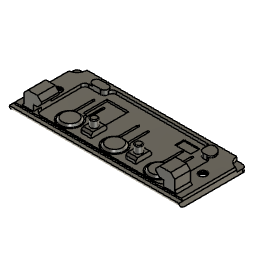
P3_Clicker (Autodesk Fusion 360 design; units mm, degrees)
Autodesk Fusion 360 part; units mm, degrees
sketch "草图1" plane through (0, 0, 0) normal (0, 0, 1) x (1, 0, 0)
  line L0 (0, 0) -> (43, 0)
  line L1 (43, 0) -> (43, 17.2)
  line L2 (43, 17.2) -> (0, 17.2)
  line L3 (0, 17.2) -> (0, 0)
  line L4 (0, 17.2) -> (3.1, 17.2) construction
  line L5 (3.1, 17.2) -> (3.1, 9.2) construction
  line L6 (3.1, 9.2) -> (0, 9.2) construction
  line L7 (0, 9.2) -> (0, 17.2) construction
  line L8 (21.5, 17.2) -> (21.5, 0) construction
  circle A0 centre (3.1, 9.2) radius 1.025
  circle A1 centre (3.1, 9.2) radius 2.05
  circle A2 centre (39.9, 9.2) radius 1.025
  circle A3 centre (39.9, 9.2) radius 2.05
  dimension "d1" = 43
  dimension "d2" = 17.2
  dimension "d17" = 3.1
  dimension "d18" = 8
  dimension "d19" = 2.05
  dimension "d20" = 4.1
  constraint horizontal L0
  constraint vertical L1
  constraint horizontal L2
  constraint vertical L3
  constraint coincident L0.start L3.end
  constraint horizontal L4
  constraint vertical L5
  constraint horizontal L6
  constraint vertical L7
  constraint midpoint L2 L8.start
  constraint midpoint L0 L8.end
  constraint coincident L5.end L6.start
  constraint concentric A0 A1
  constraint symmetric L8 A0 A2
  constraint symmetric L8 A1 A3
  measures "d1" distance of L0.start L0.end
  measures "d2" distance of L0.start L2.end
  measures "d17" distance of L2.end L4.end
  measures "d18" distance of L2.end L6.end
  measures "d19" diameter of A0
  measures "d20" diameter of A1
extrude "拉伸1" add sketch "草图1" along normal blind 1.8 contours L0 L1 L2 L3 | A0 | A1 | A2 | A3
sketch "草图2" plane through (0, 0, 1.8) normal (0, 0, 1) x (-1, 0, 0)
  line L0 (0, -17.2) -> (0, 0)
  line L1 (0, 0) -> (-43, 0)
  line L2 (-43, 0) -> (-43, -17.2)
  line L3 (-43, -17.2) -> (0, -17.2)
  circle A0 centre (0, -17.2) radius 2.5
  circle A1 centre (-43, -17.2) radius 2.5
  line L4 (0, 0) -> (-43, 0)
  line L5 (-43, 0) -> (-43, -1)
  line L6 (-43, -1) -> (0, -1)
  line L7 (0, -1) -> (0, 0)
  dimension "d5" = 5
  dimension "d6" = 5
  dimension "d11" = 1
  constraint coincident L0.start L3.end
  constraint coincident L2.end L3.start
  constraint horizontal L4
  constraint vertical L5
  constraint horizontal L6
  constraint vertical L7
  constraint coincident L0.end L1.start
  measures "d5" diameter of A0
  measures "d6" diameter of A1
  measures "d11" distance of L0.end L6.end
extrude "拉伸2" cut sketch "草图2" against normal blind 0.9 contours L0 L3 A0 | L2 L3 A1 picked at (-1.3308, -16.2037) picked at (-41.5409, -16.4033)
fillet "圆角1" radius 1 2 edges at (43, 17.2, 0.45) (0, 17.2, 0.45)
extrude "拉伸3" cut sketch "草图2" against normal blind 0.4 contours L0 L1 L2 L4 L5 L6 L7
fillet "圆角3" radius 1.5 1 edges at (21.5, 0, 0)
chamfer "倒角1" distance 0.4 angle 45 2 edges at (43, 7.85, 1.8) (0, 7.85, 1.8)
extrude "拉伸4" cut sketch "草图1" along normal up to surface (1.8 mm away) contours A0 | A2
extrude "拉伸5" cut sketch "草图1" along normal blind 0.5 contours A1 | A3
chamfer "倒角3" distance 1 angle 45 2 edges at (38.9444, 9.5707, 0.5) (2.1444, 9.5707, 0.5)
chamfer "倒角4" distance 0.2 angle 45 2 edges at (1.1887, 8.4587, 0) (37.9887, 8.4587, 0)
sketch "草图3" plane through (0, 0, 0) normal (0, 0, 1) x (1, 0, 0)
  line L0 (43, 17.2) -> (0, 17.2)
  line L1 (0, 17.2) -> (0, 0)
  line L2 (0, 0) -> (43, 0)
  line L3 (43, 0) -> (43, 17.2)
  circle A0 centre (3.1, 9.2) radius 2.05
  circle A1 centre (3.1, 9.2) radius 1.025
  circle A2 centre (39.9, 9.2) radius 2.05
  circle A3 centre (39.9, 9.2) radius 1.025
  line L4 (3.1, 9.2) -> (0, 9.2) construction
  line L5 (3.1, 17.2) -> (3.1, 9.2) construction
  line L6 (0, 9.2) -> (43, 9.2) construction
  line L7 (21.5, 16.2) -> (21.5, 18) construction
  line L8 (5.5, 9.2) -> (37.5, 9.2) construction
  line L9 (21.5, 17.2) -> (21.5, 0) construction
  line L10 (6.7892, 15.8535) -> (35.7892, 15.8535) construction
  line L11 (37.2892, 14.3535) -> (37.2892, 3.3535) construction
  line L12 (35.7892, 1.8535) -> (6.7892, 1.8535) construction
  line L13 (5.2892, 3.3535) -> (5.2892, 14.3535) construction
  line L14 (5.2892, 8.6) -> (37.2892, 8.6) construction
  line L15 (22.2892, 15.8535) -> (22.2892, 1.8535) construction
  line L16 (0, 8.6) -> (43, 8.6) construction
  arc A4 (6.7892, 15.8535) -> (5.2892, 14.3535) centre (6.7892, 14.3535) ccw construction
  arc A5 (5.2892, 3.3535) -> (6.7892, 1.8535) centre (6.7892, 3.3535) ccw construction
  arc A6 (35.7892, 1.8535) -> (37.2892, 3.3535) centre (35.7892, 3.3535) ccw construction
  arc A7 (37.2892, 14.3535) -> (35.7892, 15.8535) centre (35.7892, 14.3535) ccw construction
  arc A8 (37.7892, 14.3535) -> (35.7892, 16.3535) centre (35.7892, 14.3535) ccw
  line L17 (6.7892, 16.3535) -> (35.7892, 16.3535)
  arc A9 (6.7892, 16.3535) -> (4.7892, 14.3535) centre (6.7892, 14.3535) ccw
  line L18 (4.7892, 3.3535) -> (4.7892, 14.3535)
  arc A10 (4.7892, 3.3535) -> (6.7892, 1.3535) centre (6.7892, 3.3535) ccw
  line L19 (35.7892, 1.3535) -> (6.7892, 1.3535)
  arc A11 (35.7892, 1.3535) -> (37.7892, 3.3535) centre (35.7892, 3.3535) ccw
  line L20 (37.7892, 14.3535) -> (37.7892, 3.3535)
  point P0 (5.2892, 15.8535)
  point P1 (37.2892, 15.8535)
  point P2 (5.2892, 1.8535)
  dimension "d33" = 32
  dimension "d34" = 14
  dimension "d35" = 1.5
  dimension "d36" = 0.5
  constraint coincident L4.end L6.start
  constraint coincident L3 L6.end
  constraint perpendicular L3 L6
  constraint collinear L7 L9
  constraint horizontal L10
  constraint vertical L11
  constraint horizontal L12
  constraint vertical L13
  constraint midpoint L1 L16.start
  constraint midpoint L3 L16.end
  constraint collinear L14 L16
  constraint coincident L10 L15.start
  constraint coincident L13 L14.start
  constraint coincident P0 L10
  constraint coincident P0 L13
  constraint tangent L10 A4
  constraint tangent L13 A4
  constraint coincident L12 L15.end
  constraint coincident P2 L12
  constraint coincident P2 L13
  constraint tangent L12 A5
  constraint tangent L13 A5
  constraint equal A4 A5
  constraint coincident L11 L14.end
  constraint tangent L11 A6
  constraint tangent L12 A6
  constraint equal A4 A6
  constraint coincident P1 L10
  constraint coincident P1 L11
  constraint tangent L10 A7
  constraint tangent L11 A7
  constraint equal A4 A7
  measures "d33" distance of P0 P1
  measures "d34" distance of P0 P2
  measures "d35" radius of A4
sketch "草图4" plane through (0, 0, 1.8) normal (0, 0, 1) x (-1, 0, 0)
  circle A0 centre (-39.9, -9.2) radius 1.025
  circle A1 centre (-3.1, -9.2) radius 1.025
  line L0 (-0.4, -14.7322) -> (-0.4, -1)
  line L1 (-0.4, -1) -> (-42.6, -1)
  line L2 (-42.6, -1) -> (-42.6, -14.7322)
  arc A2 (-40.5, -17.2) -> (-42.6, -14.7322) centre (-43, -17.2) ccw
  line L3 (-40.5, -17.2) -> (-2.5, -17.2)
  arc A3 (-0.4, -14.7322) -> (-2.5, -17.2) centre (0, -17.2) ccw
  arc A4 (-37.7892, -14.3535) -> (-35.7892, -16.3535) centre (-35.7892, -14.3535) ccw
  line L4 (-37.7892, -14.3535) -> (-37.7892, -3.3535)
  arc A5 (-35.7892, -1.3535) -> (-37.7892, -3.3535) centre (-35.7892, -3.3535) ccw
  line L5 (-35.7892, -1.3535) -> (-6.7892, -1.3535)
  arc A6 (-4.7892, -3.3535) -> (-6.7892, -1.3535) centre (-6.7892, -3.3535) ccw
  line L6 (-4.7892, -3.3535) -> (-4.7892, -14.3535)
  arc A7 (-6.7892, -16.3535) -> (-4.7892, -14.3535) centre (-6.7892, -14.3535) ccw
  line L7 (-6.7892, -16.3535) -> (-35.7892, -16.3535)
  line L8 (-10.6464, -14.1527) -> (-16.1464, -14.1527)
  line L9 (-16.1464, -14.1527) -> (-16.1464, -8.1527)
  line L10 (-16.1464, -8.1527) -> (-10.6464, -8.1527)
  line L11 (-10.6464, -8.1527) -> (-10.6464, -14.1527)
  circle A8 centre (-16, -5.5) radius 0.9
  circle A9 centre (-27.3, -5.5) radius 0.9
  line L12 (-29.3027, -15.0275) -> (-33.3027, -15.0275)
  line L13 (-33.3027, -15.0275) -> (-33.3027, -12.7275)
  line L14 (-33.3027, -12.7275) -> (-29.3027, -12.7275)
  line L15 (-29.3027, -12.7275) -> (-29.3027, -15.0275)
  dimension "d39" = 5.5
  dimension "d40" = 6
  dimension "d43" = 1.8
  dimension "d44" = 1.8
  dimension "d84" = 4
  dimension "d85" = 2.3
  constraint horizontal L8
  constraint vertical L9
  constraint horizontal L10
  constraint vertical L11
  constraint horizontal L12
  constraint vertical L13
  constraint horizontal L14
  constraint vertical L15
  measures "d39" distance of L8.start L8.end
  measures "d40" distance of L8.start L10.end
  measures "d43" diameter of A8
  measures "d44" diameter of A9
  measures "d84" distance of L12.start L12.end
  measures "d85" distance of L12.start L14.end
extrude "拉伸6" cut sketch "草图4" against normal blind 0.8 contours A4 L4 A5 L5 A6 L6 A7 L7 | L8 L9 L10 L11 | A8 | A9 | L12 L13 L14 L15
sketch "草图5" plane through (0, 0, 1) normal (0, 0, 1) x (-1, 0, 0)
  line L0 (-37.7892, -3.3535) -> (-37.7892, -14.3535)
  arc A0 (-37.7892, -14.3535) -> (-35.7892, -16.3535) centre (-35.7892, -14.3535) ccw
  line L1 (-35.7892, -16.3535) -> (-6.7892, -16.3535)
  arc A1 (-6.7892, -16.3535) -> (-4.7892, -14.3535) centre (-6.7892, -14.3535) ccw
  line L2 (-4.7892, -14.3535) -> (-4.7892, -3.3535)
  arc A2 (-4.7892, -3.3535) -> (-6.7892, -1.3535) centre (-6.7892, -3.3535) ccw
  line L3 (-6.7892, -1.3535) -> (-35.7892, -1.3535)
  arc A3 (-35.7892, -1.3535) -> (-37.7892, -3.3535) centre (-35.7892, -3.3535) ccw
  line L4 (-16.1464, -8.1527) -> (-10.6464, -8.1527)
  line L5 (-10.6464, -8.1527) -> (-10.6464, -14.1527)
  line L6 (-16.1464, -14.1527) -> (-16.1464, -8.1527)
  line L7 (-10.6464, -14.1527) -> (-16.1464, -14.1527)
  circle A4 centre (-16, -5.5) radius 0.9
  circle A5 centre (-27.3, -5.5) radius 0.9
  circle A6 centre (-21.6977, -5.0059) radius 2.5
  line L8 (-20.6977, -12.0059) -> (-22.6977, -12.0059)
  line L9 (-22.6977, -12.0059) -> (-22.6977, -5.0059)
  line L10 (-22.6977, -5.0059) -> (-20.6977, -5.0059)
  line L11 (-20.6977, -5.0059) -> (-20.6977, -12.0059)
  line L12 (-20.1977, -4.5059) -> (-20.1977, -12.5059)
  line L13 (-20.1977, -12.5059) -> (-23.1977, -12.5059)
  line L14 (-23.1977, -12.5059) -> (-23.1977, -4.5059)
  line L15 (-23.1977, -4.5059) -> (-20.1977, -4.5059)
  circle A7 centre (-21.6977, -5.0059) radius 2.8
  line L16 (-31.3977, -4.5059) -> (-31.3977, -12.5059)
  line L17 (-31.3977, -12.5059) -> (-34.3977, -12.5059)
  line L18 (-34.3977, -4.5059) -> (-31.3977, -4.5059)
  line L19 (-34.3977, -12.5059) -> (-34.3977, -4.5059)
  line L20 (-31.8977, -5.0059) -> (-31.8977, -12.0059)
  line L21 (-31.8977, -12.0059) -> (-33.8977, -12.0059)
  line L22 (-33.8977, -5.0059) -> (-31.8977, -5.0059)
  line L23 (-33.8977, -12.0059) -> (-33.8977, -5.0059)
  circle A8 centre (-32.8977, -5.0059) radius 2.8
  circle A9 centre (-32.8977, -5.0059) radius 2.5
  line L24 (-11.8977, -12.5059) -> (-11.8977, -4.5059)
  line L25 (-11.8977, -4.5059) -> (-8.8977, -4.5059)
  line L26 (-8.8977, -4.5059) -> (-8.8977, -12.5059)
  line L27 (-8.8977, -12.5059) -> (-11.8977, -12.5059)
  line L28 (-11.3977, -12.0059) -> (-11.3977, -5.0059)
  line L29 (-11.3977, -5.0059) -> (-9.3977, -5.0059)
  line L30 (-9.3977, -12.0059) -> (-11.3977, -12.0059)
  line L31 (-9.3977, -5.0059) -> (-9.3977, -12.0059)
  circle A10 centre (-10.3977, -5.0059) radius 2.8
  circle A11 centre (-10.3977, -5.0059) radius 2.5
  line L32 (-9.3977, -12.0059) -> (-9.3977, -12.5059)
  line L33 (-11.3977, -12.0059) -> (-11.3977, -12.5059)
  line L34 (-22.6977, -12.0059) -> (-22.6977, -12.5059)
  line L35 (-20.6977, -12.0059) -> (-20.6977, -12.5059)
  line L36 (-33.8977, -12.0059) -> (-33.8977, -12.5059)
  line L37 (-31.8977, -12.0059) -> (-31.8977, -12.5059)
  line L38 (-33.3027, -12.7275) -> (-29.3027, -12.7275)
  line L39 (-29.3027, -12.7275) -> (-29.3027, -15.0275)
  line L40 (-33.3027, -15.0275) -> (-33.3027, -12.7275)
  line L41 (-29.3027, -15.0275) -> (-33.3027, -15.0275)
  line L42 (-14.75, -7.5) -> (-17.25, -7.5)
  line L43 (-17.25, -7.5) -> (-17.25, -3.5)
  line L44 (-17.25, -3.5) -> (-14.75, -3.5)
  line L45 (-14.75, -3.5) -> (-14.75, -7.5)
  line L46 (-14.75, -7.5) -> (-17.25, -3.5) construction
  line L47 (-17.25, -7.5) -> (-14.75, -3.5) construction
  line L48 (-28.55, -7.5) -> (-26.05, -7.5)
  line L49 (-26.05, -7.5) -> (-26.05, -3.5)
  line L50 (-26.05, -3.5) -> (-28.55, -3.5)
  line L51 (-28.55, -3.5) -> (-28.55, -7.5)
  line L52 (-28.55, -7.5) -> (-26.05, -3.5) construction
  line L53 (-26.05, -7.5) -> (-28.55, -3.5) construction
  line L54 (-4.7892, -16.3535) -> (-9.7892, -16.3535)
  line L55 (-9.7892, -16.3535) -> (-9.7892, -14.3535)
  line L56 (-9.7892, -14.3535) -> (-4.7892, -14.3535)
  line L57 (-4.7892, -14.3535) -> (-4.7892, -16.3535)
  line L58 (-37.7892, -16.3535) -> (-34.7892, -16.3535)
  line L59 (-34.7892, -16.3535) -> (-34.7892, -13.3535)
  line L60 (-34.7892, -13.3535) -> (-37.7892, -13.3535)
  line L61 (-37.7892, -13.3535) -> (-37.7892, -16.3535)
  point P0 (-16, -5.5)
  point P1 (-27.3, -5.5)
  dimension "d46" = 5
  dimension "d53" = 2
  dimension "d54" = 7
  dimension "d58" = -0.5
  dimension "d59" = 0.3
  dimension "d60" = -0.5
  dimension "d61" = 0.3
  dimension "d62" = 5
  dimension "d63" = 2
  dimension "d64" = 7
  dimension "d65" = -0.5
  dimension "d66" = 0.3
  dimension "d67" = 5
  dimension "d68" = 2
  dimension "d69" = 7
  dimension "d151" = 1.8
  dimension "d152" = 1.8
  dimension "d156" = 2.5
  dimension "d157" = 4
  dimension "d158" = 2.5
  dimension "d159" = 4
  dimension "d163" = 5
  dimension "d164" = 2
  dimension "d165" = 3
  dimension "d166" = 3
  constraint horizontal L8
  constraint vertical L9
  constraint horizontal L10
  constraint vertical L11
  constraint midpoint A6.centre L10
  constraint horizontal L21
  constraint vertical L23
  constraint horizontal L22
  constraint vertical L20
  constraint midpoint A8.centre L22
  constraint horizontal L30
  constraint vertical L28
  constraint horizontal L29
  constraint vertical L31
  constraint midpoint A10.centre L29
  constraint coincident L27 L32.end
  constraint perpendicular L27 L32
  constraint coincident L27 L33.end
  constraint perpendicular L27 L33
  constraint coincident L13 L34.end
  constraint perpendicular L13 L34
  constraint coincident L13 L35.end
  constraint perpendicular L13 L35
  constraint coincident L17 L36.end
  constraint perpendicular L17 L36
  constraint coincident L17 L37.end
  constraint perpendicular L17 L37
  constraint collinear L13 L27
  constraint collinear L13 L17
  constraint horizontal L42
  constraint perpendicular L42 L43
  constraint parallel L42 L44
  constraint parallel L43 L45
  constraint coincident L46 P0
  constraint coincident L47 P0
  constraint coincident P0 A4.centre
  constraint horizontal L48
  constraint perpendicular L48 L49
  constraint parallel L48 L50
  constraint parallel L49 L51
  constraint coincident L52 P1
  constraint coincident L53 P1
  constraint coincident P1 A5.centre
  constraint horizontal L54
  constraint vertical L55
  constraint horizontal L56
  constraint vertical L57
  constraint horizontal L58
  constraint vertical L59
  constraint horizontal L60
  constraint vertical L61
  measures "d46" diameter of A6
  measures "d53" distance of L8.start L8.end
  measures "d54" distance of L8.start L10.end
  measures "d62" diameter of A9
  measures "d63" distance of L20.end L21.end
  measures "d64" distance of L20.start L20.end
  measures "d67" diameter of A11
  measures "d68" distance of L30.start L28.start
  measures "d69" distance of L29.end L30.start
  measures "d151" diameter of A4
  measures "d152" diameter of A5
  measures "d156" distance of L43.end L44.end
  measures "d157" distance of L42.end L43.end
  measures "d158" distance of L49.end L50.end
  measures "d159" distance of L48.end L49.end
  measures "d163" distance of L54.start L54.end
  measures "d164" distance of L54.start A1.end
  measures "d165" distance of L58.start L58.end
  measures "d166" distance of L58.start L60.end
extrude "拉伸21" add sketch "草图5" along normal blind 1.2 contours L0 A0 L1 L58 L59 L60 L61 | L1 A1 L54 L55 L56
fillet "圆角9" radius 1 10 edges at (9.7892, 14.3535, 1.6) (34.7892, 13.3535, 1.6) (9.7892, 16.3535, 1.4) (4.7892, 14.3535, 1.4) (37.7892, 13.3535, 1.4) (34.7892, 16.3535, 1.4) (4.7892, 14.3535, 2) (9.7892, 16.3535, 2) (37.7892, 13.3535, 2) (34.7892, 16.3535, 2)
extrude "拉伸20" add sketch "草图5" along normal blind 1.2 contours L42 L43 L44 L45 | L48 L49 L50 L51
chamfer "倒角10" distance 0.5 angle 45 4 edges at (16, 7.5, 2.2) (16, 3.5, 2.2) (27.3, 3.5, 2.2) (27.3, 7.5, 2.2)
extrude "拉伸7" cut sketch "草图5" against normal up to surface (1 mm away) contours L4 L24 L28 A10 | L4 L24 L27 L28 L33 | L24 L26 A10 A11 | L24 L28 A10 A11 | L26 L27 L31 A10 L32 | L26 L31 A10 A11 | A6 L12 L14 A7 | A6 L9 L14 A7 | A6 L11 L12 A7 | L9 L13 L14 A7 L34 | L11 L12 L13 A7 L35 | L16 L19 A8 A9 | L16 L20 A8 A9 | L16 L17 L20 A8 L37 | L19 L23 A8 A9 | L17 L19 L23 A8 L36
extrude "拉伸9" cut sketch "草图5" against normal blind 0.5 contours L4 L5 L6 L7 L24 L27 | L4 L5 L28 L30 | L5 L27 L30 L33
extrude "拉伸11" cut sketch "草图5" against normal blind 0.3 contours L38 L39 L40 L41
extrude "拉伸10" add sketch "草图5" along normal blind 3 contours A4 | A5
fillet "圆角6" radius 0.25 12 edges at (9.3977, 12.5059, 0.5) (11.3977, 12.5059, 0.25) (22.6977, 12.5059, 0.5) (20.6977, 12.5059, 0.5) (31.8977, 12.5059, 0.5) (33.8977, 12.5059, 0.5) (31.3977, 12.5059, 0.5) (20.1977, 12.5059, 0.5) (34.3977, 12.5059, 0.5) (23.1977, 12.5059, 0.5) (11.8977, 12.5059, 0.25) (8.8977, 12.5059, 0.5)
fillet "圆角6" radius 0.75 6 edges at (34.3977, 7.3702, 0.5) (31.3977, 7.3702, 0.5) (23.1977, 7.3702, 0.5) (20.1977, 7.3702, 0.5) (11.8977, 7.3702, 0.5) (8.8977, 7.3702, 0.5)
fillet "圆角6" radius 0.3 6 edges at (11.3977, 7.2972, 0.5) (22.6977, 7.2972, 0.5) (33.8977, 7.2972, 0.5) (31.8977, 7.2972, 0.5) (20.6977, 7.2972, 0.5) (9.3977, 7.2972, 0.5)
fillet "圆角5" radius 0.2 2 edges at (28.1391, 5.8255, 4) (16.8391, 5.8255, 4)
sketch "草图6" plane through (0, 0, 0) normal (0, 0, -1) x (1, 0, 0)
  arc A0 (31.3977, -7.7518) -> (31.1231, -7.1717) centre (30.6477, -7.7518) ccw
  arc A1 (34.6724, -7.1717) -> (31.1231, -7.1717) centre (32.8977, -5.0059) ccw
  arc A2 (34.6724, -7.1717) -> (34.3977, -7.7518) centre (35.1477, -7.7518) ccw
  line L0 (34.3977, -7.7518) -> (34.3977, -12.2559)
  arc A3 (33.8977, -12.2559) -> (34.3977, -12.2559) centre (34.1477, -12.2559) ccw
  line L1 (33.8977, -12.2559) -> (33.8977, -7.4858)
  arc A4 (34.0584, -7.2201) -> (33.8977, -7.4858) centre (34.1977, -7.4858) ccw
  arc A5 (34.0584, -7.2201) -> (31.737, -7.2201) centre (32.8977, -5.0059) ccw
  arc A6 (31.8977, -7.4858) -> (31.737, -7.2201) centre (31.5977, -7.4858) ccw
  line L2 (31.8977, -7.4858) -> (31.8977, -12.2559)
  arc A7 (31.3977, -12.2559) -> (31.8977, -12.2559) centre (31.6477, -12.2559) ccw
  line L3 (31.3977, -12.2559) -> (31.3977, -7.7518)
  arc A8 (20.1977, -7.7518) -> (19.9231, -7.1717) centre (19.4477, -7.7518) ccw
  arc A9 (23.4724, -7.1717) -> (19.9231, -7.1717) centre (21.6977, -5.0059) ccw
  arc A10 (23.4724, -7.1717) -> (23.1977, -7.7518) centre (23.9477, -7.7518) ccw
  line L4 (23.1977, -7.7518) -> (23.1977, -12.2559)
  arc A11 (22.6977, -12.2559) -> (23.1977, -12.2559) centre (22.9477, -12.2559) ccw
  line L5 (22.6977, -12.2559) -> (22.6977, -7.4858)
  arc A12 (22.8584, -7.2201) -> (22.6977, -7.4858) centre (22.9977, -7.4858) ccw
  arc A13 (22.8584, -7.2201) -> (20.537, -7.2201) centre (21.6977, -5.0059) ccw
  arc A14 (20.6977, -7.4858) -> (20.537, -7.2201) centre (20.3977, -7.4858) ccw
  line L6 (20.6977, -7.4858) -> (20.6977, -12.2559)
  arc A15 (20.1977, -12.2559) -> (20.6977, -12.2559) centre (20.4477, -12.2559) ccw
  line L7 (20.1977, -12.2559) -> (20.1977, -7.7518)
  arc A16 (8.8977, -7.7518) -> (8.6231, -7.1717) centre (8.1477, -7.7518) ccw
  arc A17 (12.1724, -7.1717) -> (8.6231, -7.1717) centre (10.3977, -5.0059) ccw
  arc A18 (12.1724, -7.1717) -> (11.8977, -7.7518) centre (12.6477, -7.7518) ccw
  line L8 (11.8977, -7.7518) -> (11.8977, -12.2559)
  arc A19 (11.3977, -12.2559) -> (11.8977, -12.2559) centre (11.6477, -12.2559) ccw
  line L9 (11.3977, -12.2559) -> (11.3977, -7.4858)
  arc A20 (11.5584, -7.2201) -> (11.3977, -7.4858) centre (11.6977, -7.4858) ccw
  arc A21 (11.5584, -7.2201) -> (9.237, -7.2201) centre (10.3977, -5.0059) ccw
  arc A22 (9.3977, -7.4858) -> (9.237, -7.2201) centre (9.0977, -7.4858) ccw
  line L10 (9.3977, -7.4858) -> (9.3977, -12.2559)
  arc A23 (8.8977, -12.2559) -> (9.3977, -12.2559) centre (9.1477, -12.2559) ccw
  line L11 (8.8977, -12.2559) -> (8.8977, -7.7518)
  circle A24 centre (3.1, -9.2) radius 2.25
  line L12 (43, -1.4967) -> (0, -1.4967)
  line L13 (0, -1.4967) -> (0, -16.2)
  arc A25 (0, -16.2) -> (1, -17.2) centre (1, -16.2) ccw
  line L14 (1, -17.2) -> (42, -17.2)
  arc A26 (42, -17.2) -> (43, -16.2) centre (42, -16.2) ccw
  line L15 (43, -16.2) -> (43, -1.4967)
  circle A27 centre (39.9, -9.2) radius 2.25
  circle A28 centre (10.3977, -5.0059) radius 2.5
  circle A29 centre (21.6977, -5.0059) radius 2.5
  circle A30 centre (32.8977, -5.0059) radius 2.5
  line L16 (10.3977, -2.5059) -> (10.3977, -7.5059) construction
  line L17 (10.3977, -4.1012) -> (10.3977, -4.6012)
  circle A31 centre (10.3977, -5.0059) radius 0.75
  circle A32 centre (10.3977, -5.0059) radius 0.85
  line L18 (10.2977, -4.1012) -> (10.2977, -4.6012)
  line L19 (10.4977, -4.1012) -> (10.4977, -4.6012)
  circle A33 centre (10.3977, -5.0059) radius 0.65
  circle A34 centre (10.3977, -4.1012) radius 0.1
  circle A35 centre (10.3977, -4.6012) radius 0.1
  circle A36 centre (9.9873, -4.3781) radius 0.1
  circle A37 centre (10.8081, -4.3781) radius 0.1
  line L20 (21.6977, -2.5059) -> (21.6977, -7.5059) construction
  line L21 (21.6977, -4.2559) -> (21.6977, -5.7559)
  line L22 (21.5977, -4.2559) -> (21.5977, -5.7559)
  line L23 (21.7977, -4.2559) -> (21.7977, -5.7559)
  circle A38 centre (21.6977, -4.2559) radius 0.1
  circle A39 centre (21.6977, -5.7559) radius 0.1
  line L24 (22.4477, -4.9059) -> (20.9477, -4.9059)
  circle A40 centre (22.4477, -5.007) radius 0.1011
  line L25 (22.4477, -5.0059) -> (20.9477, -5.0059)
  circle A41 centre (20.9477, -5.007) radius 0.1011
  line L26 (33.6477, -5.0059) -> (32.1477, -5.0059)
  line L27 (33.6477, -4.9059) -> (32.1477, -4.9059)
  line L28 (33.6477, -5.1059) -> (32.1477, -5.1059)
  circle A42 centre (33.6477, -5.0059) radius 0.1
  circle A43 centre (32.1477, -5.0059) radius 0.1
  line L29 (20.9477, -5.1081) -> (22.4477, -5.1081)
  dimension "d98" = 0.5
  dimension "d99" = 1.5
  dimension "d100" = 0.1
  dimension "d101" = 0.1
  dimension "d102" = -0.1
  dimension "d103" = -0.1
  dimension "d105" = 1.5
  dimension "d106" = 0.1
  dimension "d107" = -0.1
  dimension "d113" = 0.1
  dimension "d114" = 1.5
  dimension "d115" = 1.5
  dimension "d116" = 0.1
  dimension "d117" = -0.1
  constraint midpoint A21 L16.start
  constraint coincident A28 L16.end
  constraint vertical L16
  constraint coincident L16 L17.start
  constraint parallel L16 L17
  constraint concentric A17 A31
  constraint coincident L17.start A34.centre
  constraint coincident L19.start A34
  constraint tangent L19 A34
  constraint coincident L17.end A35.centre
  constraint coincident L19.end A35
  constraint tangent L19 A35
  constraint coincident A31 A36.centre
  constraint tangent A32 A36
  constraint symmetric L16 A36 A37
  constraint midpoint A13 L20.start
  constraint coincident A29 L20.end
  constraint vertical L20
  constraint coincident L20 L21.start
  constraint parallel L20 L21
  constraint coincident L21.start A38.centre
  constraint coincident L23.start A38
  constraint tangent L23 A38
  constraint coincident L21.end A39.centre
  constraint coincident L23.end A39
  constraint tangent L23 A39
  constraint midpoint L20 L21
  constraint coincident L24.start A40
  constraint tangent L24 A40
  constraint coincident L24.end A41
  constraint tangent L24 A41
  constraint midpoint A1.centre L26
  constraint coincident L26.start A42.centre
  constraint coincident L27.start A42
  constraint tangent L27 A42
  constraint coincident L26.end A43.centre
  constraint coincident L27.end A43
  constraint tangent L27 A43
  constraint midpoint A9.centre L25
  constraint coincident A41 L29.start
  constraint coincident A40 L29.end
  constraint tangent A40 L29
  constraint perpendicular L20 L29
  measures "d98" distance of L17.start L17.end
  measures "d99" diameter of A31
  measures "d105" distance of L21.start L21.end
  measures "d114" distance of L25.start L25.end
  measures "d115" distance of L26.start L26.end
extrude "拉伸16" add sketch "草图5" along normal blind 0.5 contours L24 L25 L26 A11 | L24 L25 L26 L28 L29 L31 A11 | L28 L29 L31 A11 | A6 L12 L14 L15 | A6 L9 L10 L11 L12 L14 L15 | A6 L9 L10 L11 | L16 L18 L19 A9 | L16 L18 L19 L20 L22 L23 A9 | L20 L22 L23 A9
chamfer "倒角8" distance 0.5 angle 45 3 edges at (24.0285, 5.9099, 1.5) (12.7285, 5.9099, 1.5) (35.2285, 5.9099, 1.5)
chamfer "倒角9" distance 0.2 angle 45 36 edges at (21.6977, 2.5059, 0) (20.6544, 7.3305, 0) (20.6977, 9.8708, 0) (20.4477, 12.5059, 0) (20.1977, 10.0038, 0) (20.1256, 7.4309, 0) (21.6977, 2.2059, 0) (23.2698, 7.4309, 0) (23.1977, 10.0038, 0) (22.9477, 12.5059, 0) (22.6977, 9.8708, 0) (22.741, 7.3305, 0) (32.8977, 2.5059, 0) (31.8544, 7.3305, 0) (31.8977, 9.8708, 0) (31.6477, 12.5059, 0) (31.3977, 10.0038, 0) (31.3256, 7.4309, 0) (32.8977, 2.2059, 0) (34.4698, 7.4309, 0) (34.3977, 10.0038, 0) (34.1477, 12.5059, 0) (33.8977, 9.8708, 0) (33.941, 7.3305, 0) (10.3977, 2.5059, 0) (9.3544, 7.3305, 0) (9.3977, 9.8708, 0) (9.1477, 12.5059, 0) (8.8977, 10.0038, 0) (8.8256, 7.4309, 0) (10.3977, 2.2059, 0) (11.9698, 7.4309, 0) (11.8977, 10.0038, 0) (11.6477, 12.5059, 0) (11.3977, 9.8708, 0) (11.441, 7.3305, 0)
sketch "草图7" plane through (0, 0, 1.8) normal (0, 0, 1) x (-1, 0, 0)
  line L0 (-35.7892, -1.3535) -> (-6.7892, -1.3535)
  arc A0 (-4.7892, -3.3535) -> (-6.7892, -1.3535) centre (-6.7892, -3.3535) ccw
  line L1 (-4.7892, -3.3535) -> (-4.7892, -13.3535)
  line L2 (-10.7892, -16.3535) -> (-33.7892, -16.3535)
  line L3 (-37.7892, -12.3535) -> (-37.7892, -3.3535)
  arc A1 (-35.7892, -1.3535) -> (-37.7892, -3.3535) centre (-35.7892, -3.3535) ccw
  circle A2 centre (-39.9, -9.2) radius 1.025
  circle A3 centre (-3.1, -9.2) radius 1.025
  line L4 (-0.4, -14.7322) -> (-0.4, -1)
  line L5 (-0.4, -1) -> (-42.6, -1)
  line L6 (-42.6, -1) -> (-42.6, -14.7322)
  arc A4 (-40.5, -17.2) -> (-42.6, -14.7322) centre (-43, -17.2) ccw
  line L7 (-40.5, -17.2) -> (-2.5, -17.2)
  arc A5 (-0.4, -14.7322) -> (-2.5, -17.2) centre (0, -17.2) ccw
  line L8 (-35.7892, -1.3535) -> (-37.7892, -1.3535) construction
  line L9 (-37.7892, -3.3535) -> (-37.7892, -1.3535) construction
  line L10 (-37.7892, -1.3535) -> (-37.7891, -1.3535) construction
  line L11 (-4.7892, -1.3535) -> (-2.3892, -1.3535)
  line L12 (-2.3892, -1.3535) -> (-2.3892, -5.8535)
  line L13 (-2.3892, -5.8535) -> (-4.7892, -5.8535)
  line L14 (-4.7892, -5.8535) -> (-4.7892, -1.3535)
  line L15 (-37.7891, -1.3535) -> (-40.5891, -1.3535)
  line L16 (-40.5891, -1.3535) -> (-40.5891, -5.3535)
  line L17 (-40.5891, -5.3535) -> (-37.7891, -5.3535)
  line L18 (-37.7891, -5.3535) -> (-37.7891, -1.3535)
  line L19 (-0.4, -1.3535) -> (-8.196, -1.3535) construction
  line L20 (-2.3892, -1.3535) -> (-2.3891, -1.3535) construction
  arc A6 (-5.7892, -14.3535) -> (-4.7892, -13.3535) centre (-5.7892, -13.3535) ccw
  line L21 (-5.7892, -14.3535) -> (-6.7892, -14.3535)
  line L22 (-6.7892, -16.3535) -> (-8.7892, -16.3535)
  arc A7 (-10.7892, -16.3535) -> (-9.7892, -15.3535) centre (-10.7892, -15.3535) ccw
  arc A8 (-34.7892, -15.3535) -> (-33.7892, -16.3535) centre (-33.7892, -15.3535) ccw
  arc A9 (-37.7892, -14.3535) -> (-35.7892, -16.3535) centre (-35.7892, -14.3535) ccw
  arc A10 (-37.7892, -12.3535) -> (-36.7892, -13.3535) centre (-36.7892, -12.3535) ccw
  arc A11 (-6.7892, -16.3535) -> (-6.7892, -14.3535) centre (-6.7892, -15.3535) ccw
  arc A12 (-9.7892, -15.3535) -> (-8.7892, -16.3535) centre (-8.7892, -15.3535) ccw
  arc A13 (-35.7892, -16.3535) -> (-34.7892, -15.3535) centre (-35.7892, -15.3535) ccw
  arc A14 (-36.7892, -13.3535) -> (-37.7892, -14.3535) centre (-36.7892, -14.3535) ccw
  dimension "d128" = 2
  dimension "d131" = 2.4
  dimension "d132" = 4.5
  dimension "d133" = 2.8
  dimension "d134" = 4
  constraint coincident L0.start A1.start
  constraint parallel L0 L8
  constraint coincident L3.end A1.end
  constraint horizontal L11
  constraint vertical L12
  constraint horizontal L13
  constraint vertical L14
  constraint horizontal L15
  constraint vertical L16
  constraint horizontal L17
  constraint vertical L18
  constraint coincident L4 L19.start
  constraint coincident L0 L19.end
  constraint perpendicular L4 L19
  constraint coincident L19 L20.end
  constraint collinear L1 L14
  constraint collinear L8 L15
  constraint collinear L11 L19
  measures "d128" distance of L0.start L8.end
  measures "d131" distance of L11.start L11.end
  measures "d132" distance of L11.start L13.end
  measures "d133" distance of L10.end L15.end
  measures "d134" distance of L10.end L17.end
extrude "拉伸17" add sketch "草图7" along normal blind 4 contours L3 L15 L16 L17 L18 | L1 L11 L12 L13 L14
sketch "草图8" plane through (4.7892, 0, 0) normal (1, 0, 0) x (0, 1, 0)
  line L0 (3.3535, 1.8) -> (3.3535, 1)
  line L1 (3.3535, 1) -> (13.3535, 1)
  line L2 (13.3535, 1.8) -> (5.8535, 1.8)
  line L3 (1.3535, 5.8) -> (5.8535, 5.8)
  line L4 (5.8535, 5.8) -> (5.8535, 1.8)
  line L5 (5.8535, 1.8) -> (1.3535, 1.8)
  line L6 (1.3535, 1.8) -> (1.3535, 5.8)
  line L7 (5.8535, 1.8) -> (5.8535, 5.8)
  line L8 (5.8535, 5.8) -> (1.3535, 5.8)
  line L9 (1.3535, 5.8) -> (1.3535, 1.8)
  line L10 (1.3535, 1.8) -> (3.3535, 1.8)
  line L11 (13.3535, 1) -> (13.3535, 1.8)
  line L12 (1.3535, 1.8) -> (5.8535, 1.8) construction
  line L13 (5.8535, 1.8) -> (5.8535, 3.3) construction
  line L14 (5.8535, 3.3) -> (1.3535, 3.3) construction
  line L15 (1.3535, 3.3) -> (1.3535, 1.8) construction
  line L16 (1.3535, 5.8) -> (5.8535, 5.8)
  line L17 (5.8535, 5.8) -> (5.8535, 3.3)
  line L18 (5.8535, 3.3) -> (1.3535, 3.3)
  line L19 (1.3535, 3.3) -> (1.3535, 5.8)
  dimension "d171" = 1.5
  constraint horizontal L3
  constraint vertical L4
  constraint horizontal L5
  constraint vertical L6
  constraint coincident L2.end L4.end
  constraint collinear L6 L9
  constraint horizontal L12
  constraint vertical L13
  constraint horizontal L14
  constraint vertical L15
  constraint coincident L5.end L6.start
  constraint horizontal L16
  constraint vertical L17
  constraint horizontal L18
  constraint vertical L19
  constraint coincident L3.start L6.end
  measures "d171" distance of L5.end L14.end
extrude "拉伸22" add sketch "草图8" along normal blind 2 contours L3 L4 L6 L7 L8 L9 L16 L17 L18 L19
sketch "草图9" plane through (37.7891, 0, 0) normal (-1, 0, 0) x (0, -1, 0)
  line L0 (-3.3335, 1.8) -> (-1.3535, 1.8)
  line L1 (-1.3535, 1.8) -> (-1.3535, 5.8)
  line L2 (-1.3535, 5.8) -> (-5.3535, 5.8)
  line L3 (-5.3535, 5.8) -> (-5.3535, 1.8)
  line L4 (-5.3535, 5.8) -> (-1.3535, 5.8)
  line L5 (-1.3535, 5.8) -> (-1.3535, 1.8)
  line L6 (-1.3535, 1.8) -> (-5.3535, 1.8)
  line L7 (-5.3535, 1.8) -> (-5.3535, 5.8)
  line L8 (-5.3535, 1.8) -> (-3.3335, 1.8)
  line L9 (-1.3535, 1.8) -> (-5.3535, 1.8) construction
  line L10 (-5.3535, 1.8) -> (-5.3535, 3.3) construction
  line L11 (-5.3535, 3.3) -> (-1.3535, 3.3) construction
  line L12 (-1.3535, 3.3) -> (-1.3535, 1.8) construction
  line L13 (-5.3535, 5.8) -> (-1.3535, 5.8)
  line L14 (-1.3535, 5.8) -> (-1.3535, 3.3)
  line L15 (-1.3535, 3.3) -> (-5.3535, 3.3)
  line L16 (-5.3535, 3.3) -> (-5.3535, 5.8)
  dimension "d174" = 1.5
  constraint horizontal L4
  constraint vertical L5
  constraint horizontal L6
  constraint vertical L7
  constraint coincident L0.end L1.start
  constraint coincident L2.end L3.start
  constraint horizontal L9
  constraint vertical L10
  constraint horizontal L11
  constraint vertical L12
  constraint horizontal L13
  constraint vertical L14
  constraint horizontal L15
  constraint vertical L16
  measures "d174" distance of L0.end L11.end
extrude "拉伸23" add sketch "草图9" along normal blind 2 contours L1 L2 L3 L4 L5 L7 L13 L14 L15 L16
chamfer "倒角11" distance 1 angle 45 4 edges at (35.7891, 3.3535, 5.8) (2.3892, 3.6035, 5.8) (6.7892, 3.6035, 5.8) (40.5891, 3.3535, 5.8)
chamfer "倒角11" distance 1 angle 45 2 edges at (35.7891, 3.3535, 3.3) (6.7892, 3.6035, 3.3)
chamfer "倒角11" distance 0.5 angle 45 2 edges at (40.5891, 3.3535, 1.8) (2.3892, 3.6035, 1.8)
named bodies: "P3_Clicker"
